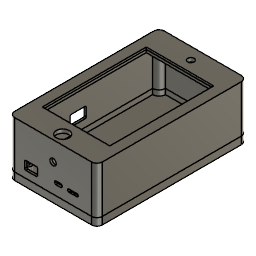
GNSS_BOX (Autodesk Fusion 360 design; units mm, degrees)
Autodesk Fusion 360 part; units mm, degrees
sketch "Sketch1" plane through (0, 0, 0) normal (0, 0, 1) x (1, 0, 0)
  line L0 (41, 70) -> (-41, 70)
  line L1 (-41, 70) -> (-41, -70)
  line L2 (-41, -70) -> (41, -70)
  line L3 (41, -70) -> (41, 70)
  line L4 (41, 70) -> (-41, -70) construction
  line L5 (-41, 70) -> (41, -70) construction
  dimension "d1" = 82
  dimension "d2" = 140
  constraint horizontal L0
  constraint perpendicular L0 L1
  constraint parallel L0 L2
  constraint parallel L1 L3
  constraint coincident L4 origin
  constraint coincident L5 origin
  measures "d1" distance of L1.end L2.end
  measures "d2" distance of L0.end L1.end
extrude "Extrude1" add sketch "Sketch1" along normal blind 2 makes body 1
sketch "Sketch2" plane through (0, 0, 2) normal (0, 0, 1) x (-1, 0, 0)
  line L0 (-41, 70) -> (-41, -70)
  line L1 (-41, -70) -> (41, -70)
  line L2 (41, -70) -> (41, 70)
  line L3 (41, 70) -> (-41, 70)
  line L4 (41, -70) -> (-41, -70)
  line L5 (-41, -70) -> (-41, 70)
  line L6 (-41, 70) -> (41, 70)
  line L7 (41, 70) -> (41, -70)
  line L8 (-39, 68) -> (39, 68)
  line L9 (39, 68) -> (39, -68)
  line L10 (39, -68) -> (-39, -68)
  line L11 (-39, -68) -> (-39, 68)
  dimension "d5" = 2
  constraint horizontal L4
  constraint vertical L5
  constraint horizontal L6
  constraint vertical L7
  constraint coincident L0.start L3.end
  constraint coincident L1.end L2.start
extrude "Extrude2" add sketch "Sketch2" along normal blind 5 bodies 1
sketch "Sketch3" plane through (0, 0, 2) normal (0, 0, 1) x (-1, 0, 0)
  line L0 (39, -68) -> (39, 68)
  line L1 (39, 68) -> (-39, 68)
  line L2 (-39, 68) -> (-39, -68)
  line L3 (-39, -68) -> (39, -68)
  circle A0 centre (-39, 68) radius 6
  circle A1 centre (-39, -68) radius 6
  circle A2 centre (39, 68) radius 6
  circle A3 centre (39, -68) radius 6
  dimension "d8" = 12
  dimension "d9" = 12
  dimension "d10" = 12
  dimension "d19" = 12
  constraint coincident L1.end L2.start
  constraint coincident L2.end L3.start
  constraint coincident L0.end L1.start
  constraint coincident L0.start L3.end
  measures "d8" diameter of A1
  measures "d9" diameter of A2
  measures "d10" diameter of A3
  measures "d19" diameter of A0
extrude "Extrude3" add sketch "Sketch3" along normal blind 5 contours L0 L3 A3 | L0 L1 A2 | L2 L3 A1 | L1 L2 A0 picked at (35.4982, -66.0879) picked at (35.0204, 67.7154) picked at (-35.1014, -67.1519) picked at (-35.0204, 67.7154) bodies 1
sketch "Sketch4" plane through (0, 0, 7) normal (0, 0, 1) x (-1, 0, 0)
  line L0 (33, -68) -> (-33, -68)
  arc A0 (-33, -68) -> (-39, -62) centre (-39, -68) ccw
  line L1 (-39, -62) -> (-39, 62)
  arc A1 (-39, 62) -> (-33, 68) centre (-39, 68) ccw
  line L2 (-33, 68) -> (33, 68)
  arc A2 (33, 68) -> (39, 62) centre (39, 68) ccw
  line L3 (39, 62) -> (39, -62)
  arc A3 (39, -62) -> (33, -68) centre (39, -68) ccw
  line L4 (41, 70) -> (-41, 70)
  line L5 (-41, 70) -> (-41, -70)
  line L6 (-41, -70) -> (41, -70)
  line L7 (41, -70) -> (41, 70)
  line L8 (-39, 68) -> (39, 68)
  line L9 (39, 68) -> (39, -68)
  line L10 (39, -68) -> (-39, -68)
  line L11 (-39, -68) -> (-39, 68)
  circle A4 centre (-37, -66) radius 1.25
  circle A5 centre (37, -66) radius 1.25
  circle A6 centre (-37, 66) radius 1.25
  circle A7 centre (37, 66) radius 1.25
  dimension "d21" = 2.5
  dimension "d23" = 2.5
  dimension "d28" = 2.5
  dimension "d29" = 2.5
  constraint horizontal L8
  constraint vertical L9
  constraint horizontal L10
  constraint vertical L11
  constraint coincident A3.centre L9.end
  constraint coincident A1.centre L8.start
  measures "d23" diameter of A5
  measures "d28" diameter of A6
  measures "d29" diameter of A7
extrude "Extrude4" cut sketch "Sketch4" against normal blind 7 contours A4 | A5 | A6 | A7 bodies 1
sketch "Sketch5" plane through (0, 0, 7) normal (0, 0, 1) x (-1, 0, 0)
  line L0 (-41, 70) -> (41, 70)
  line L1 (41, 70) -> (41, -70)
  line L2 (41, -70) -> (-41, -70)
  line L3 (-41, -70) -> (-41, 70)
  line L4 (39, -68) -> (-39, -68)
  line L5 (-39, -68) -> (-39, 68)
  line L6 (-39, 68) -> (39, 68)
  line L7 (39, 68) -> (39, -68)
  dimension "d30" = 2
  constraint horizontal L0
  constraint vertical L1
  constraint horizontal L2
  constraint vertical L3
extrude "Extrude6" add sketch "Sketch5" along normal blind 44 separate body makes body 2
sketch "Sketch7" plane through (39, 0, 0) normal (-1, 0, 0) x (0, -1, 0)
  line L0 (-68, 7) -> (68, 7)
  line L1 (68, 7) -> (68, 51)
  line L2 (68, 51) -> (-68, 51)
  line L3 (-68, 51) -> (-68, 7)
  line L4 (-68, 51) -> (68.0049, 51)
  line L5 (68.0049, 51) -> (68.0049, 49)
  line L6 (68.0049, 49) -> (-68, 49)
  line L7 (-68, 49) -> (-68, 51)
  dimension "d41" = 2
  constraint horizontal L4
  constraint vertical L5
  constraint horizontal L6
  constraint vertical L7
  constraint coincident L2.end L3.start
  measures "d41" distance of L2.end L6.end
extrude "Extrude7" add sketch "Sketch7" along normal blind 78 contours L1 L4 L5 L6 bodies 2
sketch "Sketch8" plane through (0, 0, 7) normal (0, 0, 1) x (-1, 0, 0)
  circle A0 centre (39, 68) radius 6
  circle A1 centre (-39, 68) radius 6
  circle A2 centre (-39, -68) radius 6
  circle A3 centre (39, -68) radius 6
  line L0 (39, 68) -> (-39, 68)
  line L1 (-39, 68) -> (-39, -68)
  line L2 (-39, -68) -> (39, -68)
  line L3 (39, -68) -> (39, 68)
  dimension "d44" = 12
  dimension "d45" = 12
  dimension "d46" = 12
  dimension "d47" = 12
  constraint horizontal L0
  constraint vertical L1
  constraint horizontal L2
  constraint vertical L3
  constraint coincident A2.centre L1.end
  constraint coincident A0.centre L0.start
  measures "d44" diameter of A0
  measures "d45" diameter of A1
  measures "d46" diameter of A2
  measures "d47" diameter of A3
extrude "Extrude8" add sketch "Sketch4" sketch "Sketch8" along normal blind 44 contours A0 L10 L11 of sketch 2 contours A0 L0 L3 | A1 L0 L1 | A3 L2 L3 picked at (35.0204, 67.7154) picked at (-35.1014, 67.1519) picked at (35.0204, -67.7154) bodies 2
sketch "Sketch9" plane through (0, 0, 7) normal (0, 0, 1) x (-1, 0, 0)
  circle A0 centre (37, -66) radius 1.25
  circle A1 centre (-37, -66) radius 1.25
  circle A2 centre (37, 66) radius 1.25
  circle A3 centre (-37, 66) radius 1.25
  dimension "d50" = 2.5
  dimension "d51" = 2.5
  dimension "d52" = 2.5
  dimension "d53" = 2.5
  measures "d50" diameter of A0
  measures "d51" diameter of A1
  measures "d52" diameter of A2
  measures "d53" diameter of A3
sketch "Sketch11" plane through (39, 0, 0) normal (-1, 0, 0) x (0, -1, 0)
  line L0 (-62, 51) -> (-62, 7)
  line L1 (-62, 7) -> (62, 7)
  line L2 (62, 7) -> (62, 51)
  line L3 (62, 51) -> (-62, 51)
  line L4 (-68, 51) -> (68, 51)
  line L5 (68, 51) -> (68, 47.5)
  line L6 (68, 47.5) -> (-68, 47.5)
  line L7 (-68, 47.5) -> (-68, 51)
  dimension "d60" = 3.5
  constraint horizontal L4
  constraint vertical L5
  constraint horizontal L6
  constraint vertical L7
  measures "d60" distance of L4.start L6.end
extrude "Extrude11" add sketch "Sketch11" along normal blind 78 contours L0 L2 L3 L4 L6 | L0 L4 L6 L7 | L2 L4 L5 L6 bodies 2
extrude "Extrude12" cut sketch "Sketch9" along normal blind 20 bodies 2
sketch "Sketch12" plane through (0, 0, 0) normal (0, 0, -1) x (1, 0, 0)
  circle A0 centre (37, -66) radius 1.25
  circle A1 centre (-37, 66) radius 1.25
  circle A2 centre (-37, -66) radius 1.25
  circle A3 centre (37, 66) radius 1.25
  line L0 (41, -70) -> (41, 70)
  line L1 (41, 70) -> (-41, 70)
  line L2 (-41, 70) -> (-41, -70)
  line L3 (-41, -70) -> (41, -70)
  circle A4 centre (37, -66) radius 2.25
  circle A5 centre (-37, -66) radius 2.25
  circle A6 centre (37, 66) radius 2.25
  circle A7 centre (-37, 66) radius 2.25
  dimension "d65" = 4.5
  dimension "d66" = 4.5
  dimension "d67" = 4.5
  dimension "d68" = 4.5
  constraint concentric A0 A4
  constraint concentric A2 A5
  constraint concentric A3 A6
  constraint concentric A1 A7
  measures "d66" diameter of A5
  measures "d67" diameter of A6
  measures "d68" diameter of A7
extrude "Extrude13" cut sketch "Sketch12" against normal blind 1.2 contours A0 | A1 | A2 | A3 | A4 | A5 | A6 | A7 bodies 1
sketch "Sketch13" plane through (0, 0, 51) normal (0, 0, 1) x (-1, 0, 0)
  line L0 (-41, -70) -> (41, -70)
  line L1 (41, -70) -> (41, 70)
  line L2 (41, 70) -> (-41, 70)
  line L3 (-41, 70) -> (-41, -70)
  line L4 (30.5, 47.5) -> (-30.5, 47.5)
  line L5 (-30.5, 47.5) -> (-30.5, -47.5)
  line L6 (-30.5, -47.5) -> (30.5, -47.5)
  line L7 (30.5, -47.5) -> (30.5, 47.5)
  line L8 (30.5, 47.5) -> (-30.5, -47.5) construction
  line L9 (-30.5, 47.5) -> (30.5, -47.5) construction
  dimension "d71" = 61
  dimension "d72" = 95
  constraint horizontal L4
  constraint perpendicular L4 L5
  constraint parallel L4 L6
  constraint parallel L5 L7
  constraint coincident L8 origin
  constraint coincident L9 origin
  measures "d71" distance of L5.end L6.end
  measures "d72" distance of L4.end L5.end
extrude "Extrude14" cut sketch "Sketch13" against normal blind 3.5 contours L4 L5 L6 L7 bodies 2
sketch "Sketch14" plane through (0, 0, 51) normal (0, 0, 1) x (-1, 0, 0)
  line L0 (-30.5, 47.5) -> (30.5, 47.5)
  line L1 (30.5, 47.5) -> (30.5, -47.5)
  line L2 (30.5, -47.5) -> (-30.5, -47.5)
  line L3 (-30.5, -47.5) -> (-30.5, 47.5)
  line L4 (-41, -70) -> (41, -70)
  line L5 (41, -70) -> (41, 70)
  line L6 (41, 70) -> (-41, 70)
  line L7 (-41, 70) -> (-41, -70)
  line L8 (-30.5, -47.5) -> (30.5, -47.5)
  line L9 (30.5, -47.5) -> (30.5, -70)
  line L10 (30.5, -70) -> (-30.5, -70)
  line L11 (-30.5, -70) -> (-30.5, -47.5)
  circle A0 centre (0, -58.75) radius 3
  line L12 (-30.5, 47.5) -> (30.5, 47.5)
  line L13 (30.5, 47.5) -> (30.5, 70)
  line L14 (30.5, 70) -> (-30.5, 70)
  line L15 (-30.5, 70) -> (-30.5, 47.5)
  circle A1 centre (0, 61) radius 6
  dimension "d75" = 6
  dimension "d78" = 12
  constraint horizontal L8
  constraint vertical L9
  constraint horizontal L10
  constraint vertical L11
  constraint coincident L4 L9.end
  constraint coincident L2.end L3.start
  constraint horizontal L12
  constraint vertical L13
  constraint horizontal L14
  constraint vertical L15
  constraint coincident L6 L13.end
  constraint coincident L0.start L3.end
  measures "d75" diameter of A0
  measures "d78" diameter of A1
extrude "Extrude15" cut sketch "Sketch14" against normal blind 3.5 contours A0 | A1 bodies 2
sketch "Sketch15" plane through (0, 0, 2) normal (0, 0, 1) x (-1, 0, 0)
  arc A0 (39, -62) -> (33, -68) centre (39, -68) ccw
  line L0 (39, -62) -> (39, 62)
  arc A1 (33, 68) -> (39, 62) centre (39, 68) ccw
  line L1 (33, 68) -> (-33, 68)
  arc A2 (-39, 62) -> (-33, 68) centre (-39, 68) ccw
  line L2 (-39, 62) -> (-39, -62)
  arc A3 (-33, -68) -> (-39, -62) centre (-39, -68) ccw
  line L3 (-33, -68) -> (33, -68)
  line L4 (32.5, -68) -> (-32.5, -68)
  line L5 (32.5, -68) -> (32.5, -37.5)
  line L6 (32.5, -37.5) -> (-32.5, -37.5)
  line L7 (-32.5, -37.5) -> (-32.5, -68)
  line L8 (32.5, -68) -> (29, -68)
  line L9 (29, -68) -> (29, -64.5) construction
  line L10 (29, -64.5) -> (32.5, -64.5) construction
  line L11 (32.5, -64.5) -> (32.5, -68)
  circle A4 centre (29, -64.5) radius 1.25
  line L12 (0, -68) -> (0, -37.5) construction
  line L13 (32.5, -37.5) -> (29, -37.5)
  line L14 (29, -37.5) -> (29, -41) construction
  line L15 (29, -41) -> (32.5, -41) construction
  line L16 (32.5, -41) -> (32.5, -37.5)
  circle A5 centre (29, -41) radius 1.25
  circle A6 centre (29, -64.5) radius 3.25
  circle A7 centre (29, -41) radius 3.25
  circle A8 centre (-29, -64.5) radius 3.25
  circle A9 centre (-29, -64.5) radius 1.25
  circle A10 centre (-29, -41) radius 3.25
  circle A11 centre (-29, -41) radius 1.25
  line L17 (39, 0) -> (-39, 0) construction
  line L18 (32.5, 68) -> (-32.5, 68)
  circle A12 centre (-29, 41) radius 1.25
  circle A13 centre (-29, 64.5) radius 3.25
  circle A14 centre (29, 64.5) radius 3.25
  line L19 (32.5, 68) -> (29, 68)
  line L20 (32.5, 64.5) -> (32.5, 68)
  circle A15 centre (29, 64.5) radius 1.25
  circle A16 centre (29, 41) radius 1.25
  line L21 (29, 64.5) -> (32.5, 64.5) construction
  line L22 (29, 68) -> (29, 64.5) construction
  circle A17 centre (29, 41) radius 3.25
  line L23 (32.5, 41) -> (32.5, 37.5)
  line L24 (29, 41) -> (32.5, 41) construction
  line L25 (32.5, 37.5) -> (-32.5, 37.5)
  line L26 (32.5, 68) -> (32.5, 37.5)
  circle A18 centre (-29, 41) radius 3.25
  circle A19 centre (-29, 64.5) radius 1.25
  line L27 (-33, 68) -> (33, 68)
  line L28 (32.5, 37.5) -> (29, 37.5)
  line L29 (-32.5, 37.5) -> (-32.5, 68)
  line L30 (0, 68) -> (0, 37.5) construction
  line L31 (29, 37.5) -> (29, 41) construction
  arc A20 (-39, 62) -> (-33, 68) centre (-39, 68) ccw
  arc A21 (33, 68) -> (39, 62) centre (39, 68) ccw
  point P0 (0, -68)
  point P1 (0, 68)
  dimension "d79" = 65
  dimension "d80" = 30.5
  dimension "d81" = 3.5
  dimension "d82" = 3.5
  dimension "d83" = 2.5
  dimension "d85" = 3.5
  dimension "d86" = 2.5
  dimension "d87" = 2
  dimension "d88" = 2
  constraint midpoint L4 P0
  constraint coincident L3 P0
  constraint parallel L3 L4
  constraint perpendicular L4 L5
  constraint perpendicular L5 L6
  constraint perpendicular L4 L7
  constraint horizontal L8
  constraint vertical L9
  constraint horizontal L10
  constraint vertical L11
  constraint coincident L9.end L10.start
  constraint coincident P0 L12.start
  constraint midpoint L6 L12.end
  constraint horizontal L13
  constraint vertical L14
  constraint horizontal L15
  constraint vertical L16
  constraint coincident L14.end L15.start
  constraint symmetric A4 L12 A9
  constraint symmetric L12 A5 A11
  constraint symmetric L12 A6 A8
  constraint symmetric L12 A7 A10
  constraint midpoint L0 L17.start
  constraint midpoint L2 L17.end
  constraint symmetric A0.start L17 L0.end
  constraint symmetric A0.end L17 A1.start
  constraint symmetric A0 L17 A21
  constraint symmetric L2.end L17 A2.start
  constraint symmetric A3.start L17 L1.end
  constraint symmetric A3 L17 A20
  constraint symmetric L4.start L17 L18.start
  constraint symmetric L4.end L17 L18.end
  constraint symmetric P0 L17 P1
  constraint symmetric L5.end L17 L23.end
  constraint symmetric L6.end L17 L25.end
  constraint symmetric L8.end L17 L19.end
  constraint symmetric L9.end L17 A14.centre
  constraint symmetric L10.end L17 L20.start
  constraint symmetric A4 L17 A15
  constraint symmetric L12.end L17 L30.end
  constraint symmetric L13.end L17 L28.end
  constraint symmetric L14.end L17 A16.centre
  constraint symmetric L15.end L17 L23.start
  constraint symmetric A5 L17 A16
  constraint symmetric A6 L17 A14
  constraint symmetric A7 L17 A17
  constraint symmetric A8 L17 A13
  constraint symmetric A9 L17 A19
  constraint symmetric A10 L17 A18
  constraint symmetric A11 L17 A12
  measures "d79" distance of L4.start L4.end
  measures "d80" distance of L4.start L5.end
  measures "d81" distance of L4.start L8.end
  measures "d82" distance of L4.start L10.end
  measures "d83" diameter of A4
  measures "d85" distance of L5.end L15.end
  measures "d86" diameter of A5
extrude "Extrude16" add sketch "Sketch15" along normal blind 12 contours A13 | A14 | A17 | A18 bodies 1
sketch "Sketch16" plane through (0, -70, 0) normal (0, 1, 0) x (-1, 0, 0)
  line L0 (-41, 0) -> (41, 0)
  line L1 (41, 0) -> (41, 7)
  line L2 (41, 7) -> (-41, 7)
  line L3 (-41, 7) -> (-41, 0)
  line L4 (-41, 7) -> (41, 7)
  line L5 (41, 7) -> (41, 25)
  line L6 (41, 25) -> (-41, 25)
  line L7 (-41, 25) -> (-41, 7)
  line L8 (0, 25) -> (0, 7) construction
  line L9 (-32.5, 14) -> (32.5, 14)
  line L10 (-32.5, 14) -> (-32.5, 16)
  line L11 (-32.5, 16) -> (32.5, 16)
  line L12 (32.5, 16) -> (32.5, 14)
  line L13 (32.5, 16) -> (-32.5, 16)
  line L14 (-32.5, 16) -> (-32.5, 19)
  line L15 (-32.5, 19) -> (32.5, 19)
  line L16 (32.5, 19) -> (32.5, 16)
  line L17 (32.5, 19) -> (25.5, 19)
  line L18 (25.5, 19) -> (15.5, 19)
  line L19 (15.5, 19) -> (15.5, 16)
  line L20 (15.5, 16) -> (25.5, 16)
  line L21 (25.5, 16) -> (25.5, 19)
  line L22 (15.5, 16) -> (-1.5, 16)
  line L23 (-1.5, 16) -> (-8.5, 16)
  line L24 (-8.5, 16) -> (-8.5, 19)
  line L25 (-8.5, 19) -> (-1.5, 19)
  line L26 (-1.5, 19) -> (-1.5, 16)
  line L27 (26.5, 13.5) -> (14.5, 13.5)
  line L28 (14.5, 13.5) -> (14.5, 21.5)
  line L29 (14.5, 21.5) -> (26.5, 21.5)
  line L30 (26.5, 21.5) -> (26.5, 13.5)
  line L31 (26.5, 13.5) -> (14.5, 21.5) construction
  line L32 (14.5, 13.5) -> (26.5, 21.5) construction
  line L33 (-41, 25) -> (-8.5, 25)
  line L34 (-8.5, 25) -> (-8.5, 7)
  line L35 (-8.5, 7) -> (-41, 7)
  line L36 (-41, 7) -> (-41, 25)
  line L37 (-8.5, 14) -> (-13.5, 14)
  line L38 (-13.5, 16) -> (-23.5, 16)
  line L39 (-23.5, 16) -> (-23.5, 19)
  line L40 (-23.5, 19) -> (-13.5, 19)
  line L41 (-13.5, 19) -> (-13.5, 16)
  line L42 (-23.5, 18.5) -> (-13.5, 18.5)
  line L43 (-13.5, 16) -> (-15.5, 16)
  line L44 (-15.5, 16) -> (-16.5, 16)
  line L45 (-16.5, 16) -> (-18.5, 16)
  line L46 (-18.5, 16) -> (-19.5, 16)
  line L47 (-19.5, 16) -> (-21.5, 16)
  line L48 (-21.5, 16) -> (-22.5, 16)
  line L49 (-41, 51) -> (41, 51)
  line L50 (41, 51) -> (41, 7)
  line L51 (41, 7) -> (-41, 7)
  line L52 (-41, 7) -> (-41, 51)
  circle A0 centre (0, 33) radius 3
  line L53 (41, 7) -> (-41, 7)
  line L54 (-41, 7) -> (-41, 51)
  line L55 (-41, 51) -> (41, 51)
  line L56 (41, 51) -> (41, 7)
  point P0 (0, 14)
  point P1 (20.5, 17.5)
  dimension "d91" = 65
  dimension "d92" = 2
  dimension "d93" = 3
  dimension "d94" = 7
  dimension "d95" = 10
  dimension "d96" = 3
  dimension "d97" = 17
  dimension "d98" = 7
  dimension "d99" = 8
  dimension "d102" = 5
  dimension "d103" = 10
  dimension "d104" = 3
  dimension "d119" = 6
  constraint horizontal L4
  constraint vertical L5
  constraint horizontal L6
  constraint vertical L7
  constraint coincident L2.end L3.start
  constraint midpoint L6 L8.start
  constraint midpoint L4 L8.end
  constraint midpoint L9 P0
  constraint coincident L8 P0
  constraint perpendicular L8 L9
  constraint perpendicular L9 L10
  constraint perpendicular L10 L11
  constraint horizontal L13
  constraint vertical L14
  constraint horizontal L15
  constraint vertical L16
  constraint perpendicular L16 L17
  constraint horizontal L18
  constraint vertical L19
  constraint horizontal L20
  constraint vertical L21
  constraint coincident L11 L22.end
  constraint horizontal L23
  constraint vertical L24
  constraint horizontal L25
  constraint vertical L26
  constraint coincident L15 L24.end
  constraint horizontal L27
  constraint perpendicular L27 L28
  constraint parallel L27 L29
  constraint parallel L28 L30
  constraint coincident L31 P1
  constraint coincident L32 P1
  constraint horizontal L33
  constraint vertical L34
  constraint horizontal L35
  constraint vertical L36
  constraint coincident L4 L34.end
  constraint coincident L9 L37.start
  constraint coincident L34 L37.start
  constraint coincident L9 L37.end
  constraint horizontal L38
  constraint vertical L39
  constraint horizontal L40
  constraint vertical L41
  constraint coincident L13 L38.start
  constraint coincident L39 L42.start
  constraint coincident L41 L42.end
  constraint perpendicular L41 L42
  constraint coincident L11 L43.end
  constraint coincident L38 L44.end
  constraint midpoint L38 L45.end
  constraint coincident L38 L46.end
  constraint coincident L38 L47.end
  constraint coincident L38 L48.end
  constraint horizontal L49
  constraint vertical L50
  constraint horizontal L51
  constraint vertical L52
  constraint coincident L1.end L2.start
  measures "d91" distance of L9.start L9.end
  measures "d92" distance of L9.start L10.end
  measures "d93" distance of L11.end L15.end
  measures "d94" distance of L15.end L17.end
  measures "d95" distance of L17.end L18.end
  measures "d96" distance of L17.end L20.end
  measures "d97" distance of L19.end L22.end
  measures "d98" distance of L22.end L23.end
  measures "d99" distance of L27.end L28.end
  measures "d102" distance of L37.start L37.end
  measures "d103" distance of L38.start L38.end
  measures "d104" distance of L38.start L40.end
  measures "d119" diameter of A0
extrude "Extrude17" cut sketch "Sketch16" along normal blind 2 contours L9 L11 L13 L20 L22 L28 L30 | L9 L27 L28 L30 | L11 L13 L15 L23 L24 L25 L26 L34 | L11 L13 L15 L19 L22 L28 | L11 L13 L38 L39 L41 L42 L43 L44 L45 L46 L47 L48 | L11 L13 L15 L17 L21 L30 | L11 L13 L15 L18 L19 L20 L21 | L15 L17 L18 L28 L29 L30 | A0 bodies 2
sketch "Sketch17" plane through (-41, 0, 0) normal (-1, 0, 0) x (0, -1, 0)
  line L0 (-70, 7) -> (70, 7)
  line L1 (70, 7) -> (70, 51)
  line L2 (70, 51) -> (-70, 51)
  line L3 (-70, 51) -> (-70, 7)
  line L4 (47.5, 51) -> (-47.5, 51) construction
  line L5 (-47.5, 51) -> (7.5, 51) construction
  line L6 (7.5, 51) -> (7.5, 7) construction
  line L7 (7.5, 51) -> (7.5, 24) construction
  line L8 (7.5, 24) -> (7.5, 14) construction
  line L9 (0, 24) -> (15, 24)
  line L10 (0, 14) -> (15, 14)
  line L11 (15, 24) -> (15, 14)
  line L12 (0, 24) -> (0, 14)
  line L13 (-47.5, 51) -> (-26.5, 51)
  line L14 (-26.5, 51) -> (0.5, 51)
  line L15 (-26.5, 51) -> (-26.5, 46) construction
  line L16 (-26.5, 46) -> (-26.5, 42)
  line L17 (-26.5, 42) -> (2.5, 42)
  line L18 (2.5, 42) -> (2.5, 46)
  line L19 (2.5, 46) -> (-26.5, 46)
  line L20 (0, 42) -> (0, 24) construction
  point P0 (0, 51)
  dimension "d111" = 95
  dimension "d112" = 55
  dimension "d113" = 27
  dimension "d114" = 10
  dimension "d115" = 15
  dimension "d116" = 15
  dimension "d132" = 21
  dimension "d133" = 27
  dimension "d136" = 5
  dimension "d137" = 29
  dimension "d138" = 4
  constraint midpoint L4 P0
  constraint coincident L2 P0
  constraint coincident L2 L4.end
  constraint coincident L4 L5.end
  constraint coincident L0 L6.end
  constraint perpendicular L0 L6
  constraint coincident L6 L7.end
  constraint coincident L6 L8.end
  constraint midpoint L7.end L9
  constraint perpendicular L8 L9
  constraint midpoint L8.end L10
  constraint perpendicular L6 L10
  constraint parallel L5 L13
  constraint coincident L4 L14.end
  constraint perpendicular L5 L15
  constraint perpendicular L5 L16
  constraint perpendicular L7 L17
  constraint perpendicular L17 L18
  constraint perpendicular L16 L19
  constraint coincident L17 L20.start
  constraint perpendicular L9 L20
  measures "d111" distance of L4.start L4.end
  measures "d112" distance of L4.end L5.end
  measures "d113" distance of L5.end L7.end
  measures "d114" distance of L7.end L8.end
  measures "d115" distance of L9.start L9.end
  measures "d116" distance of L10.start L10.end
  measures "d132" distance of L4.end L13.end
  measures "d133" distance of L13.end L14.end
  measures "d136" distance of L13.end L15.end
  measures "d137" distance of L16.end L17.end
  measures "d138" distance of L15.end L16.end
extrude "Extrude18" cut sketch "Sketch17" against normal blind 2 contours L9 L10 L11 L12 | L16 L17 L18 L19 bodies 2
fillet "Fillet1" radius 1 24 edges at (-26.5, -69, 21.5) (-14.5, -69, 21.5) (-26.5, -69, 13.5) (-14.5, -69, 13.5) (8.5, -69, 16) (8.5, -69, 19) (1.5, -69, 16) (1.5, -69, 19) (13.5, -69, 18.5) (23.5, -69, 18.5) (13.5, -69, 16) (23.5, -69, 16) (-40, -15, 24) (-40, 0, 24) (-40, -15, 14) (-40, 0, 14) (30.5, 0, 51) (0, -47.5, 51) (-30.5, 0, 51) (0, 47.5, 51) (-40, 26.5, 46) (-40, -2.5, 46) (-40, 26.5, 42) (-40, -2.5, 42) on bodies 2
fillet "Fillet2" radius 5 8 edges at (-41, -70, 3.5) (41, -70, 3.5) (-41, 70, 3.5) (41, 70, 3.5) (-41, -70, 29) (41, -70, 29) (-41, 70, 29) (41, 70, 29) on bodies 1 2
sketch "Sketch18" plane through (0, 0, 47.5) normal (0, 0, -1) x (1, 0, 0)
  circle A0 centre (0, -58.75) radius 3
  circle A1 centre (0, 61) radius 6
  line L0 (-30.5, 47.5) -> (30.5, 47.5)
  line L1 (30.5, 47.5) -> (30.5, -47.5)
  line L2 (30.5, -47.5) -> (-30.5, -47.5)
  line L3 (-30.5, -47.5) -> (-30.5, 47.5)
  arc A2 (-33, -68) -> (-39, -62) centre (-39, -68) ccw
  line L4 (-33, -68) -> (33, -68)
  arc A3 (39, -62) -> (33, -68) centre (39, -68) ccw
  line L5 (39, -62) -> (39, 62)
  arc A4 (33, 68) -> (39, 62) centre (39, 68) ccw
  line L6 (33, 68) -> (-33, 68)
  arc A5 (-39, 62) -> (-33, 68) centre (-39, 68) ccw
  line L7 (-39, 62) -> (-39, -62)
  line L8 (-30.5, 47.5) -> (30.5, 47.5)
  line L9 (30.5, 47.5) -> (30.5, -47.5)
  line L10 (30.5, -47.5) -> (-30.5, -47.5)
  line L11 (-30.5, -47.5) -> (-30.5, 47.5)
  line L12 (-30.5, 47.5) -> (-30.5, 51) construction
  line L13 (-30.5, 51) -> (-27.8, 51) construction
  circle A6 centre (-27.8, 51) radius 1.25
  line L14 (30.5, 47.5) -> (30.5, 51) construction
  line L15 (30.5, 51) -> (27.8, 51) construction
  circle A7 centre (27.8, 51) radius 1.25
  line L16 (-30.5, 0) -> (30.5, 0) construction
  circle A8 centre (-27.8, -51) radius 1.25
  circle A9 centre (27.8, -51) radius 1.25
  dimension "d124" = 3.5
  dimension "d125" = 2.7
  dimension "d126" = 2.5
  dimension "d127" = 3.5
  dimension "d128" = 2.7
  dimension "d129" = 2.5
  constraint horizontal L8
  constraint vertical L9
  constraint horizontal L10
  constraint vertical L11
  constraint coincident L1.end L2.start
  constraint coincident L0.start L3.end
  constraint perpendicular L8 L12
  constraint perpendicular L12 L13
  constraint coincident L13.end A6.centre
  constraint perpendicular L8 L14
  constraint perpendicular L14 L15
  constraint coincident L15.end A7.centre
  constraint midpoint L11 L16.start
  constraint midpoint L9 L16.end
  constraint symmetric A6 L16 A8
  constraint symmetric A7 L16 A9
  measures "d124" distance of L0.start L12.end
  measures "d125" distance of L12.end L13.end
  measures "d126" diameter of A6
  measures "d127" distance of L0.end L14.end
  measures "d128" distance of L14.end L15.end
  measures "d129" diameter of A7
extrude "Extrude19" cut sketch "Sketch18" against normal blind 2 contours A6 | A7 | A8 | A9 bodies 2
named bodies: "Bottom", "Top"
